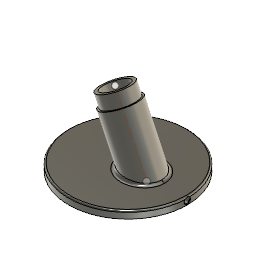
alkane-lamp-plate-v5 (Autodesk Fusion 360 design; units mm, degrees)
Autodesk Fusion 360 part; units mm, degrees
sketch "Skizze13" plane through (0, 0, 0) normal (0, 0, 1) x (1, 0, 0)
  circle A0 centre (0, 0) radius 80
extrude "Extrusion17" add sketch "Skizze13" along normal blind 10 makes body 1
fillet "Abrundung5" radius 2 1 edges at (-74.5862, -28.9292, 10) on bodies 1
sketch "Skizze14" plane through (0, 0, 0) normal (0, 1, 0) x (1, 0, 0)
  line L0 (25, 0) -> (-17.2618, -90.6308) construction
ref_plane "Arbeitsebene5" through (-17.2618, 0, 90.6308) normal (-0.422618, 0, 0.906308) x (0, -1, 0)
sketch "Skizze15" plane through (-17.2618, 0, 90.6308) normal (-0.422618, 0, 0.906308) x (0, -1, 0)
  circle A0 centre (0, 0) radius 24
  circle A1 centre (0, 0) radius 21.5
extrude "Extrusion20" add sketch "Skizze15" against normal blind 110 separate body contours A0 | A1 makes body 2
combine "Kombinieren3" operation add target body 1 tool bodies 2
extrude "Extrusion21" cut sketch "Skizze15" against normal blind 17 bodies 1
fillet "Abrundung6" radius 4 1 edges at (46.818, 0, 10) on bodies 1
sketch "Skizze16" plane through (-17.2618, 0, 90.6308) normal (-0.422618, 0, 0.906308) x (0, -1, 0)
  circle A0 centre (0, 0) radius 17
extrude "Extrusion22" cut sketch "Skizze16" against normal blind 160 bodies 1
sketch "Skizze17" plane through (0, 0, 0) normal (0, 0, 1) x (1, 0, 0)
  circle A0 centre (0, 0) radius 160
extrude "Extrusion23" cut sketch "Skizze17" against normal blind 110 bodies 1
ref_plane "Arbeitsebene6" through (90, 0, 0) normal (1, 0, 0) x (0, 1, 0)
sketch "Skizze18" plane through (90, 0, 0) normal (1, 0, 0) x (0, 0, -1)
  circle A0 centre (-5, 0) radius 3.5
extrude "Extrusion24" cut sketch "Skizze18" against normal blind 70 bodies 1
chamfer "Fase3" distance 0.7 angle 45 3 edges at (41.122, -3.4937, 4.7932) (79.9365, 0.0176, 8.5) (80, 0, 1.5) on bodies 1
equation "base_plate_diameter = 160 mm" comment "Durchmesser der runden Basis-Platte"
equation "base_plate_height = 10 mm" comment "Höhe der runden Basis-Platte"
equation "base_plate_rounding = 2 mm" comment "Abrundung der oberen Basis-Platte-Kante"
equation "arm_outer_diameter = 48 mm" comment "Aussendurchmesser des Fußbeines"
equation "ring_inner_diameter = 43 mm" comment "Aussendurchmesser des oberen Anschluss-Steckzapfens"
equation "ring_extrude_depth = 17 mm" comment "Länge des oberen Anschluss-Steckzapfens / Stufenabsatzes"
equation "foot_leg_bore_diameter = 34 mm" comment "Innendurchmesser des Beins / Kabeldurchführung (34mm)"
equation "leg_length = 100 mm" comment "Länge des Beins von der Basis-Platte zum oberen Anschluss"
equation "leg_angle = 115 deg" comment "Winkel des Beines zur Basis-Platte"
equation "leg_offset = 25 mm" comment "Abstand des Bein-Fußpunktes vom Plattenmittelpunkt"
equation "leg_plate_rounding = 4 mm" comment "Abrundung der Kante zwischen Bein und Basis-Platte"
equation "cable_hole_offset = 90 mm" comment "Versatz der Kabelkanal-Konstruktionsebene"
equation "cable_hole_depth = 70 mm" comment "Schnitttiefe des Kabelkanals (70mm)"
equation "cable_hole_diameter = 7 mm" comment "Durchmesser des Kabelkanallochs"
equation "cable_hole_height = 5.0 mm" comment "Höhe des Kabelkanallochs über der Unterseite"
equation "cable_hole_chamfer = 0.7 mm" comment "Abfasung der Lochkanten des Kabelkanals"
equation "d81 = base_plate_height"
equation "d84 = base_plate_rounding"
equation "d90 = -leg_length - base_plate_height"
equation "d92 = -ring_extrude_depth"
equation "d95 = leg_plate_rounding"
equation "d96 = -leg_length - base_plate_height - 50 mm"
equation "d102 = -cable_hole_depth"
equation "d104 = cable_hole_chamfer"
named bodies: "Plate_Foot"
